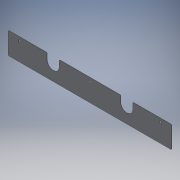
# Autodesk Inventor part: wiper 2
Saved by Autodesk Inventor 2019 (Build 230136000, 136)
## iProperties
Created: 2020-07-09
Part Number: wiper 2
Material: Generic
Document SubType Name: Modeling
Designer: Vijay
Density: 1 g/cm^3
Appearance: Default
Author: Vijay
Autodesk Inventor part; units mm, degrees
ref_plane "YZ Plane" through (0, 0, 0) normal (1, 0, 0) x (0, 1, 0)
ref_plane "XZ Plane" through (0, 0, 0) normal (0, 1, 0) x (-1, 0, 0)
ref_plane "XY Plane" through (0, 0, 0) normal (0, 0, 1) x (1, 0, 0)
sketch "Sketch1" plane through (0, 0, 0) normal (0, 0, 1) x (1, 0, 0)
  circle A0 centre (0, 4) radius 2 construction
  circle A1 centre (-195, 4) radius 2 construction
  circle A2 centre (195, 4) radius 2 construction
  arc A3 (213, -12) -> (215, -10) centre (213, -10) ccw construction
  line L0 (215, -10) -> (215, 10) construction
  arc A4 (215, 10) -> (213, 12) centre (213, 10) ccw construction
  line L1 (213, 12) -> (-213, 12) construction
  line L2 (94, -2.8) -> (94, -7.2) construction
  line L3 (94, -7.2) -> (87.6, -7.2) construction
  line L4 (87.6, -7.2) -> (87.6, -2.8) construction
  line L5 (87.6, -2.8) -> (94, -2.8) construction
  line L6 (-108.8, -2.8) -> (-108.8, -7.2) construction
  line L7 (-108.8, -7.2) -> (-115.2, -7.2) construction
  line L8 (-115.2, -7.2) -> (-115.2, -2.8) construction
  line L9 (-115.2, -2.8) -> (-108.8, -2.8) construction
  line L10 (115.2, -2.8) -> (115.2, -7.2) construction
  line L11 (115.2, -7.2) -> (108.8, -7.2) construction
  line L12 (108.8, -7.2) -> (108.8, -2.8) construction
  line L13 (108.8, -2.8) -> (115.2, -2.8) construction
  line L14 (-87.6, -2.8) -> (-87.6, -7.2) construction
  line L15 (-87.6, -7.2) -> (-94, -7.2) construction
  line L16 (-94, -7.2) -> (-94, -2.8) construction
  line L17 (-94, -2.8) -> (-87.6, -2.8) construction
  circle A5 centre (-101.4, -5) radius 1.6 construction
  circle A6 centre (101.4, -5) radius 1.6 construction
  line L18 (213.9083, -46) -> (-214.0917, -46) construction
  line L19 (-225, 12) -> (225, 12)
  line L20 (225, 12) -> (225, -46)
  line L21 (-225, -46) -> (-225, 12)
  line L22 (-225, -46) -> (225, -46)
  line L23 (197, -54.5741) -> (193, -54.5741)
  line L24 (2, -54.5741) -> (-2, -54.5741)
  line L25 (-195, -54.5741) -> (-197, -54.5741)
  line L26 (-108.8, -54.5741) -> (-115.2, -54.5741)
  line L27 (94, -54.5741) -> (87.6, -54.5741)
  line L28 (-225, -46) -> (225, -46)
  line L29 (225, -46) -> (225, -48)
  line L30 (225, -48) -> (-225, -48)
  line L31 (-225, -48) -> (-225, -46)
  line L32 (-195, 4) -> (-195, 0) construction
  line L33 (-197, 4) -> (-197, 0)
  line L34 (-193, 0) -> (-193, 4)
  arc A7 (-193, 4) -> (-197, 4) centre (-195, 4) ccw
  arc A8 (-197, 0) -> (-193, 0) centre (-195, 0) ccw
  line L35 (0, 4) -> (0, 0) construction
  line L36 (-2, 4) -> (-2, 0)
  line L37 (2, 0) -> (2, 4)
  arc A9 (2, 4) -> (-2, 4) centre (0, 4) ccw
  arc A10 (-2, 0) -> (2, 0) centre (0, 0) ccw
  line L38 (195, 4) -> (195, 0) construction
  line L39 (193, 4) -> (193, 0)
  line L40 (197, 0) -> (197, 4)
  arc A11 (197, 4) -> (193, 4) centre (195, 4) ccw
  arc A12 (193, 0) -> (197, 0) centre (195, 0) ccw
  circle A13 centre (0, 4) radius 2 construction
  circle A14 centre (-195, 4) radius 2 construction
  circle A15 centre (195, 4) radius 2 construction
  arc A16 (213, -12) -> (215, -10) centre (213, -10) ccw construction
  line L41 (215, -10) -> (215, 10) construction
  arc A17 (215, 10) -> (213, 12) centre (213, 10) ccw construction
  line L42 (213, 12) -> (-213, 12) construction
  arc A18 (-213, 12) -> (-215, 10) centre (-213, 10) ccw construction
  line L43 (-215, 10) -> (-215, -10) construction
  arc A19 (-215, -10) -> (-213, -12) centre (-213, -10) ccw construction
  line L44 (-213, -12) -> (213, -12) construction
  line L45 (94, -2.8) -> (94, -7.2) construction
  line L46 (94, -7.2) -> (87.6, -7.2) construction
  line L47 (87.6, -7.2) -> (87.6, -2.8) construction
  line L48 (87.6, -2.8) -> (94, -2.8) construction
  line L49 (-108.8, -2.8) -> (-108.8, -7.2) construction
  line L50 (-108.8, -7.2) -> (-115.2, -7.2) construction
  line L51 (-115.2, -7.2) -> (-115.2, -2.8) construction
  line L52 (-115.2, -2.8) -> (-108.8, -2.8) construction
  line L53 (115.2, -2.8) -> (115.2, -7.2) construction
  line L54 (115.2, -7.2) -> (108.8, -7.2) construction
  line L55 (108.8, -7.2) -> (108.8, -2.8) construction
  line L56 (108.8, -2.8) -> (115.2, -2.8) construction
  line L57 (-87.6, -2.8) -> (-87.6, -7.2) construction
  line L58 (-87.6, -7.2) -> (-94, -7.2) construction
  line L59 (-94, -7.2) -> (-94, -2.8) construction
  line L60 (-94, -2.8) -> (-87.6, -2.8) construction
  circle A20 centre (-101.4, -5) radius 1.6 construction
  circle A21 centre (101.4, -5) radius 1.6 construction
  point P0 (-213, -12)
  point P1 (-195, 2)
  point P2 (0, 2)
  point P3 (195, 2)
  dimension "d0" = 2
  dimension "d1" = 58
  dimension "d5" = 4
  dimension "d6" = 4
  dimension "d7" = 4
  dimension "d17" = 10
  dimension "d18" = 10
  constraints: 52 end point, 14 point on circle, 12 parallel, 12 tangent, 7 centre point, 4 point on line, 3 concentric, 3 horizontal, 3 midpoint, 2 collinear, 2 perpendicular, 1 vertical
  measures "d0" distance of L28.end L29.end
  measures "d1" distance of L19.end L20.end
  measures "d5" distance of L32.start L32.end
  measures "d6" distance of L35.start L35.end
  measures "d7" distance of L38.start L38.end
  measures "d17" distance between parallel lines of L21 L43
  measures "d18" distance between parallel lines of L0 L20
extrude "Extrusion2" add sketch "Sketch1" along normal blind 1
fillet "Fillet2" radius 2 4 edges at (-225, -48, 0.5) (-225, 12, 0.5) (225, 12, 0.5) (225, -48, 0.5)
sketch "Sketch2" plane through (0, 0, 1) normal (0, 0, 1) x (1, 0, 0)
  circle A0 centre (-101.4, -5) radius 1.6 projected
  circle A1 centre (101.4, -5) radius 1.6 projected
  line L0 (115, -3) -> (115, -7) projected
  line L1 (87.6, -7.2) -> (87.6, -2.8) projected
  line L2 (-87.8, -3) -> (-87.8, -7) projected
  line L3 (-115, -3) -> (-115, -7) projected
  line L4 (-101.4, 24.0788) -> (-101.4, -5) construction
  line L5 (-118.4, 24.0788) -> (-118.4, -5)
  line L6 (-84.4, -5) -> (-84.4, 24.0788)
  arc A2 (-84.4, 24.0788) -> (-118.4, 24.0788) centre (-101.4, 24.0788) ccw
  arc A3 (-118.4, -5) -> (-84.4, -5) centre (-101.4, -5) ccw
  line L7 (101.4, 38.8521) -> (101.4, -5) construction
  line L8 (84.4, 38.8521) -> (84.4, -5)
  line L9 (118.4, -5) -> (118.4, 38.8521)
  arc A4 (118.4, 38.8521) -> (84.4, 38.8521) centre (101.4, 38.8521) ccw
  arc A5 (84.4, -5) -> (118.4, -5) centre (101.4, -5) ccw
  point P0 (-101.4, 9.5394)
  point P1 (101.4, 16.926)
  dimension "d13" = 17
  constraints: 16 end point, 8 point on circle, 8 tangent, 4 centre point, 3 parallel, 2 midpoint, 1 equal radius, 1 vertical
  measures "d13" radius of A4
extrude "Extrusion3" cut sketch "Sketch2" against normal blind 1 contours A0 | A1 | A2 L6 A3 L5 | A4 L9 A5 L8
fillet "Fillet3" radius 2 4 edges at (-118.4, 12, 0.5) (-84.4, 12, 0.5) (84.4, 12, 0.5) (118.4, 12, 0.5)
body "Solid2"
